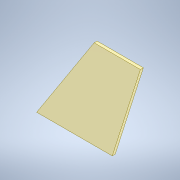
# Autodesk Inventor part: fin set
Saved by Autodesk Inventor 2020 (Build 240168000, 168)
## iProperties
Created: 2022-02-17
Part Number: fin set
Material: Generic
Document SubType Name: Modeling
Designer: User
Density: 1 g/cm^3
Appearance: Nylon 6
Author: User
Autodesk Inventor part; units mm, degrees
ref_plane "YZ Plane" through (0, 0, 0) normal (1, 0, 0) x (0, 1, 0)
ref_plane "XZ Plane" through (0, 0, 0) normal (0, 1, 0) x (-1, 0, 0)
ref_plane "XY Plane" through (0, 0, 0) normal (0, 0, 1) x (1, 0, 0)
sketch "Sketch1" plane through (0, 0, 0) normal (0, 0, 1) x (1, 0, 0)
  line L0 (10.364, 14.0947) -> (41.5508, 14.0947)
  line L1 (22.5763, -45.9053) -> (-28.4492, -45.9053)
  line L2 (41.5508, 14.0947) -> (22.5763, -45.9053)
  line L3 (-28.4492, -45.9053) -> (10.364, 14.0947)
  point P0 (0, 0)
  constraints: 8 end point, 1 horizontal, 1 parallel
extrude "Extrusion1" add sketch "Sketch1" along normal blind 2
body "Solid1"
